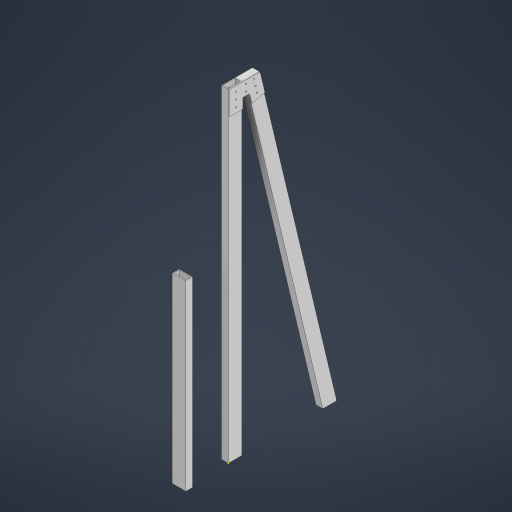
# Autodesk Inventor part: Truss
Saved by Autodesk Inventor 2023 (Build 270158000, 158)
## iProperties
Created: 2023-01-10
Part Number: Truss
Material: Generic
Document SubType Name: Modeling
Designer: Terrence
Density: 1 g/cm^3
Appearance: Default
Author: Terrence
Autodesk Inventor part; units mm, degrees
ref_plane "YZ Plane" through (0, 0, 0) normal (1, 0, 0) x (0, 1, 0)
ref_plane "XZ Plane" through (0, 0, 0) normal (0, 1, 0) x (-1, 0, 0)
ref_plane "XY Plane" through (0, 0, 0) normal (0, 0, 1) x (1, 0, 0)
sketch "Sketch1" plane through (0, 0, 0) normal (0, 1, 0) x (-1, 0, 0)
  line L0 (0, 0) -> (-25.4, 0)
  line L1 (-25.4, 0) -> (-25.4, -50.8)
  line L2 (-25.4, -50.8) -> (0, -50.8)
  line L3 (0, -50.8) -> (0, 0)
  dimension "d0" = 25.4
  dimension "d1" = 50.8
  constraints: 8 end point, 2 parallel, 1 horizontal, 1 perpendicular
  measures "d0" distance of L2.end L1.end
  measures "d1" distance of L1.end L0.end
extrude "Extrusion1" add sketch "Sketch1" along normal blind 1219.2
shell "Shell1" thickness 3.175 removed faces 2 at (16.9333, 1219.2, -33.8667) at (16.9333, 0, -33.8667)
sketch "Sketch2" plane through (25.4, 0, 0) normal (1, 0, 0) x (0, 0, -1)
  line L0 (50.8, 1219.2) -> (0, 1219.2) construction
  line L1 (116.2844, 1219.2) -> (407.8323, 0)
  line L2 (50.8, 0) -> (50.8, 1219.2) construction
  line L3 (50.8, 0) -> (407.8323, 0) construction
  line L4 (76.2, 1168.4) -> (355.6, 0)
  line L5 (0, 1219.2) -> (50.8, 1219.2) projected
  line L6 (355.6, 0) -> (407.8323, 0)
  line L7 (50.8, 0) -> (50.8, 1219.2) projected
  line L8 (50.8, 1219.2) -> (101.6, 1219.2)
  line L9 (101.6, 1219.2) -> (257.7199, 1219.2) construction
  line L10 (50.8, 1168.4) -> (76.2, 1168.4)
  line L11 (101.6, 1219.2) -> (116.2844, 1219.2)
  line L12 (76.2, 1168.4) -> (116.2844, 1219.2)
  point P0 (0, 0)
  dimension "d5" = 357.0323
  dimension "d6" = 50.8
  dimension "d21" = 304.8
  dimension "d22" = 50.8
  dimension "d23" = 50.8
  dimension "d24" = 25.4
  constraints: 18 end point, 4 horizontal, 2 point on line, 1 collinear, 1 parallel, 2 other
  measures "d5" distance of L2.start L1.end
  measures "d6" distance between parallel lines of L1 L4
  measures "d21" distance of L4.end L2.start
  measures "d22" distance of L0.start L8.end
  measures "d23" distance between parallel lines of L8 L10
  measures "d24" distance of L10.start L4.start
extrude "Extrusion2" add sketch "Sketch2" against normal blind 25.4 separate body contours L1 L6 L4 L12
ref_plane "Work Plane1" through (0, 0, -407.8323) normal (0, -0.9725789, -0.2325732) x (1, 0, 0)
sketch "Sketch3" plane through (0, 0, -407.8323) normal (0, -0.9725789, -0.2325732) x (1, 0, 0)
  line L0 (0, 0) -> (0, 50.8) projected
  line L1 (25.4, 0) -> (0, 0) projected
  line L2 (25.4, 50.8) -> (25.4, 0) projected
  line L3 (25.4, 50.8) -> (0, 50.8) projected
  line L4 (3.175, 47.625) -> (3.175, 3.175)
  line L5 (3.175, 3.175) -> (22.225, 3.175)
  line L6 (22.225, 3.175) -> (22.225, 47.625)
  line L7 (22.225, 47.625) -> (3.175, 47.625)
  point P0 (0, 396.6491)
  dimension "d9" = 3.175
  constraints: 8 end point, 3 other
  measures "d9" distance between parallel lines of L0 L4
extrude "Extrusion3" cut sketch "Sketch3" against normal blind 1452.5625 contours L7 L6 L5 L4 bodies 2
sketch "Sketch6" plane through (25.4, 0, 0) normal (1, 0, 0) x (0, 0, -1)
  point P0 (0, 0)
sketch "Sketch7" plane through (0, 0, 0) normal (0, 1, 0) x (-1, 0, 0)
  line L0 (-36.7303, 171.5828) -> (14.0697, 171.5828)
  line L1 (14.0697, 171.5828) -> (14.0697, 146.1828)
  line L2 (14.0697, 146.1828) -> (-36.7303, 146.1828)
  line L3 (-36.7303, 146.1828) -> (-36.7303, 171.5828)
  point P0 (0, 0)
  dimension "d16" = 50.8
  dimension "d17" = 25.4
  constraints: 8 end point, 2 parallel, 1 horizontal, 1 perpendicular
  measures "d16" distance of L1.end L2.end
  measures "d17" distance of L0.end L1.end
extrude "Extrusion4" add sketch "Sketch7" along normal blind 685.8 separate body
shell "Shell2" thickness 3.175 removed faces 2 at (19.7969, 685.8, 163.1161) at (19.7969, 0, 163.1161) bodies 3
extrude "Extrusion5" add sketch "Sketch2" against normal blind 25.4 separate body contours L12 L10 L7 L8 L11
ref_plane "Work Plane2" through (25.4, 1219.2, -116.2844) normal (0, 0, -1) x (-1, 0, 0)
sketch "Sketch8" plane through (25.4, 1219.2, -116.2844) normal (0, 0, -1) x (-1, 0, 0)
  line L0 (0, -50.8) -> (0, 0) projected
  line L1 (0, -50.8) -> (25.4, -50.8) projected
  line L2 (25.4, 0) -> (25.4, -50.8) projected
  line L3 (0, 0) -> (25.4, 0) projected
  line L4 (22.225, -47.625) -> (3.175, -47.625)
  line L5 (3.175, -47.625) -> (3.175, -3.175)
  line L6 (3.175, -3.175) -> (22.225, -3.175)
  line L7 (22.225, -3.175) -> (22.225, -47.625)
  point P0 (25.4, -1219.2)
  dimension "d27" = 3.175
  constraints: 8 end point, 3 other
  measures "d27" distance between parallel lines of L2 L7
extrude "Extrusion6" cut sketch "Sketch8" against normal blind 139.7 contours L4 L5 L6 L7 bodies 4
sketch "Sketch9" plane through (25.4, 0, 0) normal (1, 0, 0) x (0, 0, -1)
  line L0 (50.8, 0) -> (50.8, 1219.2) projected
  line L1 (50.8, 1130.3) -> (0, 1130.3)
  line L2 (0, 1130.3) -> (0, 1219.2)
  line L3 (76.2, 1168.4) -> (50.8, 1168.4) projected
  line L4 (50.8, 1130.3) -> (50.8, 1168.4)
  line L5 (50.8, 1168.4) -> (76.2, 1168.4)
  line L6 (76.2, 1168.4) -> (85.061, 1131.3447)
  line L7 (358.8645, 0) -> (78.7053, 1171.575) projected
  line L8 (85.061, 1131.3447) -> (134.468, 1143.1595)
  line L9 (407.8323, 0) -> (116.2844, 1219.2) projected
  line L10 (116.2844, 1219.2) -> (76.2, 1168.4) projected
  line L11 (116.2844, 1219.2) -> (134.468, 1143.1595)
  line L12 (0, 0) -> (0, 1219.2) projected
  line L13 (50.8, 1219.2) -> (116.2844, 1219.2) projected
  line L14 (0, 1219.2) -> (116.2844, 1219.2)
  point P0 (88.149, 1132.0832)
  dimension "d30" = 88.9
  dimension "d31" = 38.1
  constraints: 16 end point, 3 perpendicular, 2 collinear, 2 point on line, 1 parallel
  measures "d30" distance between parallel lines of L14 L1
  measures "d31" distance of L3.start L6.end
extrude "Extrusion7" add sketch "Sketch9" along normal blind 3.175 separate body
sketch "Sketch10" plane through (28.575, 0, 0) normal (1, 0, 0) x (0, 0, -1)
  line L0 (50.8, 1168.4) -> (76.2, 1168.4) projected
  line L1 (63.5, 1168.4) -> (63.5, 1219.2) construction
  line L2 (116.2844, 1219.2) -> (0, 1219.2) projected
  circle A0 centre (63.5, 1206.5) radius 2.667
  circle A1 centre (63.5, 1181.1) radius 2.667
  line L3 (85.061, 1131.3447) -> (134.468, 1143.1595) projected
  line L4 (109.7645, 1137.2521) -> (90.1683, 1219.2) construction
  line L5 (25.4, 1122.68) -> (25.4, 1218.3533) construction
  circle A2 centre (25.4, 1200.15) radius 2.667
  circle A3 centre (25.4, 1149.35) radius 2.667
  circle A4 centre (25.4, 1174.75) radius 2.667
  line L6 (0, 1130.3) -> (50.8, 1130.3) projected
  circle A5 centre (104.9367, 1157.4412) radius 2.667
  circle A6 centre (93.122, 1206.8482) radius 2.667
  circle A7 centre (99.0293, 1182.1447) radius 2.667
  point P0 (0, 0)
  point P1 (25.4, 1130.3)
  dimension "d34" = 5.334
  dimension "d35" = 12.7
  dimension "d36" = 12.7
  dimension "d37" = 5.334
  dimension "d38" = 5.334
  dimension "d39" = 5.334
  dimension "d40" = 19.05
  dimension "d41" = 25.4
  dimension "d42" = 25.4
  dimension "d45" = 5.334
  dimension "d46" = 5.334
  dimension "d47" = 5.334
  dimension "d48" = 12.7
  dimension "d49" = 25.4
  dimension "d50" = 25.4
  constraints: 11 point on line, 8 centre point, 6 end point, 3 midpoint, 2 perpendicular, 1 equal radius, 1 vertical
  measures "d34" diameter of A0
  measures "d35" distance from line of L0 A1.centre
  measures "d36" distance from line of L2 A0.centre
  measures "d37" diameter of A2
  measures "d38" diameter of A3
  measures "d39" diameter of A4
  measures "d40" distance from line of L2 A2.centre
  measures "d41" distance of A2.centre A4.centre
  measures "d42" distance of A4.centre A3.centre
  measures "d45" diameter of A5
  measures "d46" diameter of A6
  measures "d47" diameter of A7
  measures "d48" distance of L4.end A6.centre
  measures "d49" distance of A6.centre A7.centre
  measures "d50" distance of A5.centre A7.centre
extrude "Extrusion8" cut sketch "Sketch10" against normal through all bodies 5 1 4 2
fillet "Fillet1" radius 3.175 2 edges at (26.9875, 1168.4, -50.8) (26.9875, 1168.4, -76.2)
fillet "Fillet1" radius 3.175 6 edges at (26.9875, 1130.3, 0) (26.9875, 1219.2, 0) (26.9875, 1219.2, -116.2844) (26.9875, 1143.1595, -134.468) (26.9875, 1131.3447, -85.061) (26.9875, 1130.3, -50.8)
body "Solid1"
body "Solid2"
body "Solid3"
body "Solid4"
body "Solid5"
